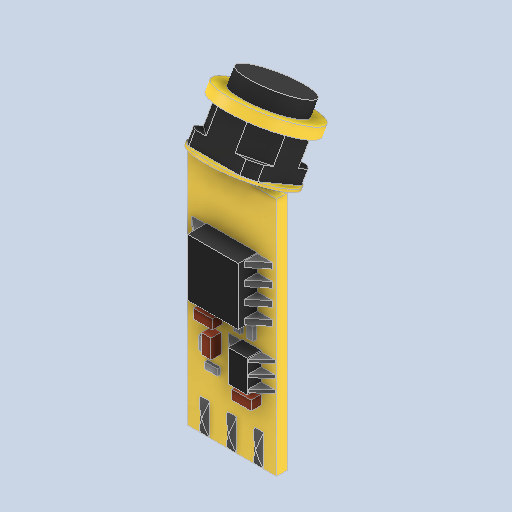
# Autodesk Inventor part: PScaled Modelart2
Saved by Autodesk Inventor 2026.2 (Build 302298010, 298A)
## iProperties
Created: 2026-05-05
Part Number: PScaled Modelart2
Material: Generic
Document SubType Name: Modeling
Designer: piete
Density: 1 g/cm^3
Appearance: Gray
Author: piete
Autodesk Inventor part; units mm, degrees
sketch "Sketch1" plane through (0, 0, 0) normal (1, 0, 0) x (0, 1, 0)
  line L0 (10.261, 0.445) -> (-8.629, 0.445)
  line L1 (-8.629, 0.445) -> (-8.629, -0.445)
  line L2 (-8.629, -0.445) -> (10.261, -0.445)
  line L3 (10.261, -0.445) -> (10.261, 0.445)
  point P0 (0, 0)
  dimension "d0" = 18.89
  dimension "d1" = 0.89
  dimension "d2" = 0.445
  dimension "d3" = 8.629
  constraints: 8 end point, 2 parallel, 1 horizontal, 1 perpendicular
  measures "d0" distance of L2.end L1.end
  measures "d1" distance of L0.end L1.end
  measures "d2" distance from line of point (0, 0) L2
  measures "d3" distance from line of L1 point (0, 0)
extrude "Extrusion1" add sketch "Sketch1" along normal blind 7
sketch "Sketch7" plane through (0, -8.629, 0.445) normal (0, 0, 1) x (1, 0, 0)
  line L0 (1.5, 14.5) -> (5.5, 14.5)
  line L1 (5.5, 14.5) -> (5.5, 10)
  line L2 (5.5, 10) -> (1.5, 10)
  line L3 (1.5, 10) -> (1.5, 14.5)
  line L4 (7, 18.89) -> (7, 0) projected
  line L5 (0, 0) -> (7, 0) projected
  point P0 (0, 8.629)
  dimension "d55" = 4
  dimension "d56" = 1.5
  dimension "d57" = 10
  dimension "d58" = 4.5
  constraints: 8 end point, 2 parallel, 1 horizontal, 1 perpendicular
  measures "d55" distance of L0.start L0.end
  measures "d56" distance between parallel lines of L4 L1
  measures "d57" distance between parallel lines of L5 L2
  measures "d58" distance of L0.end L1.end
extrude "Extrusion7" add sketch "Sketch7" along normal blind 1.5
sketch "Sketch8" plane through (1.5, 5.871, 0.445) normal (0, 1, 0) x (1, 0, 0)
  line L0 (-1.5, 0) -> (5.5, 0) projected
  line L1 (0, 0) -> (-1.2, 0)
  line L2 (0, 0) -> (0, -1)
  line L3 (0, -1) -> (-1.2, 0)
  line L4 (-1.5, 0.89) -> (-1.5, 0) projected
  point P0 (-1.5, 0.445)
  dimension "d61" = 1.2
  dimension "d62" = 1
  dimension "d63" = 0.3
  constraints: 6 end point, 2 point on line, 1 perpendicular
  measures "d61" distance of L1.start L1.end
  measures "d62" distance of L1.start L2.end
  measures "d63" distance from line of L4 L1.end
extrude "Extrusion8" add sketch "Sketch8" against normal up to surface (4.5 mm away)
sketch "Sketch9" plane through (0, -8.629, 1.945) normal (0, 0, 1) x (1, 0, 0)
  line L0 (0.3, 10) -> (0.3, 14.5) projected
  line L1 (1.5, 14.5) -> (1.5, 10) projected
  line L2 (0.3, 14.5) -> (1.5, 14.5)
  line L3 (1.5, 14.5) -> (1.5, 14.425)
  line L4 (1.5, 14.425) -> (0.3, 14.425)
  line L5 (0.3, 14.425) -> (0.3, 14.5)
  line L6 (0.3, 13.975) -> (1.5, 13.975)
  line L7 (1.5, 13.975) -> (1.5, 13.125)
  line L8 (1.5, 13.125) -> (0.3, 13.125)
  line L9 (0.3, 13.125) -> (0.3, 13.975)
  line L10 (0.3, 12.675) -> (1.5, 12.675)
  line L11 (1.5, 12.675) -> (1.5, 11.825)
  line L12 (1.5, 11.825) -> (0.3, 11.825)
  line L13 (0.3, 11.825) -> (0.3, 12.675)
  line L14 (0.3, 11.375) -> (1.5, 11.375)
  line L15 (1.5, 11.375) -> (1.5, 10.525)
  line L16 (1.5, 10.525) -> (0.3, 10.525)
  line L17 (0.3, 10.525) -> (0.3, 11.375)
  line L18 (0.3, 10) -> (1.5, 10) projected
  line L19 (0.3, 10.075) -> (1.5, 10.075)
  line L20 (1.5, 10.075) -> (1.5, 10)
  line L21 (1.5, 10) -> (0.3, 10)
  line L22 (0.3, 10) -> (0.3, 10.075)
  point P0 (0, 8.629)
  point P1 (0.3, 11.825)
  dimension "d66" = 1.2
  dimension "d67" = 1.2
  dimension "d68" = 1.2
  dimension "d69" = 0.075
  dimension "d70" = 0.075
  dimension "d71" = 0.45
  dimension "d72" = 0.45
  dimension "d73" = 0.45
  dimension "d74" = 0.45
  dimension "d75" = 0.85
  dimension "d76" = 0.85
  constraints: 40 end point, 10 parallel, 5 horizontal, 5 perpendicular, 5 point on line
  measures "d66" distance of L7.end L8.end
  measures "d67" distance of L11.end L12.end
  measures "d68" distance of L15.end L16.end
  measures "d69" distance between parallel lines of L18 L19
  measures "d70" distance between parallel lines of L2 L4
  measures "d71" distance between parallel lines of L4 L6
  measures "d72" distance between parallel lines of L10 L8
  measures "d73" distance between parallel lines of L14 L12
  measures "d74" distance between parallel lines of L19 L16
  measures "d75" distance between parallel lines of L8 L6
  measures "d76" distance between parallel lines of L12 L10
extrude "Extrusion9" cut sketch "Sketch9" against normal up to surface (1.5 mm away) contours L0 L19 L1 L18 | L0 L14 L1 L16 | L0 L10 L1 L12 | L0 L6 L1 L8 | L0 L2 L1 L4
ref_plane "Work Plane1" through (3.5, 0, 0) normal (-1, 0, 0) x (0, 0, 1)
mirror "Mirror1" about plane through (3.5, 0, 0) normal (-1, 0, 0) of "Extrusion8", "Extrusion9"
sketch "Sketch10" plane through (0, -8.629, 0.445) normal (0, 0, 1) x (1, 0, 0)
  line L0 (4.3, 5.5) -> (5.8, 5.5)
  line L1 (5.8, 5.5) -> (5.8, 8)
  line L2 (5.8, 8) -> (4.3, 8)
  line L3 (4.3, 8) -> (4.3, 5.5)
  line L4 (7, 18.89) -> (7, 0) projected
  line L5 (1.5, 10) -> (5.5, 10) projected
  point P0 (0, 8.629)
  dimension "d79" = 1.5
  dimension "d80" = 2.5
  dimension "d81" = 1.2
  dimension "d82" = 2
  constraints: 8 end point, 2 parallel, 1 horizontal, 1 perpendicular
  measures "d79" distance of L2.end L1.end
  measures "d80" distance of L1.end L0.end
  measures "d81" distance between parallel lines of L4 L1
  measures "d82" distance between parallel lines of L5 L2
extrude "Extrusion10" add sketch "Sketch10" along normal blind 1.1
sketch "Sketch11" plane through (4.3, -3.129, 0.445) normal (0, -1, 0) x (1, 0, 0)
  line L0 (1.5, 0) -> (1.5, 1.1) projected
  line L1 (1.5, 0) -> (2.6, 0)
  line L2 (1.2, 0) -> (2.4, 0) projected
  line L3 (1.5, 0) -> (2.6, 0) construction
  line L4 (1.5, 0) -> (1.5, 1)
  line L5 (1.5, 1) -> (2.6, 0)
  point P0 (-4.3, -0.445)
  point P1 (2.6, 0)
  dimension "d85" = 1.1
  dimension "d86" = 0
  dimension "d87" = 1
  constraints: 8 end point, 2 collinear, 1 horizontal, 1 point on line
  measures "d85" distance of L0.start L1.end
  measures "d86" distance between parallel lines of L1 L3
  measures "d87" distance of L0.start L4.end
extrude "Extrusion11" add sketch "Sketch11" against normal up to surface (2.5 mm away)
sketch "Sketch12" plane through (0, -8.629, 1.545) normal (0, 0, 1) x (1, 0, 0)
  line L0 (5.8, 5.5) -> (5.8, 8) projected
  line L1 (5.8, 7.9) -> (6.9, 7.9)
  line L2 (6.9, 7.9) -> (6.9, 7.65)
  line L3 (6.9, 7.65) -> (5.8, 7.65)
  line L4 (5.8, 7.65) -> (5.8, 7.9)
  line L5 (5.8, 6.875) -> (6.9, 6.875)
  line L6 (6.9, 6.875) -> (6.9, 6.625)
  line L7 (6.9, 6.625) -> (5.8, 6.625)
  line L8 (5.8, 6.625) -> (5.8, 6.875)
  line L9 (5.8, 5.85) -> (6.9, 5.85)
  line L10 (6.9, 5.85) -> (6.9, 5.6)
  line L11 (6.9, 5.6) -> (5.8, 5.6)
  line L12 (5.8, 5.6) -> (5.8, 5.85)
  line L13 (6.9, 5.5) -> (5.8, 5.5) projected
  line L14 (6.9, 8) -> (5.8, 8) projected
  line L15 (4.3, 5.5) -> (5.8, 5.5) projected
  line L16 (6.9, 8) -> (6.9, 5.5) projected
  line L17 (5.8, 8) -> (6.9, 8)
  line L18 (6.9, 8) -> (6.9, 5.5)
  line L19 (6.9, 5.5) -> (5.8, 5.5)
  line L20 (5.8, 5.5) -> (5.8, 8)
  point P0 (0, 8.629)
  point P1 (6.9, 6.75)
  dimension "d90" = 1.1
  dimension "d91" = 0.25
  dimension "d92" = 1.1
  dimension "d93" = 0.25
  dimension "d94" = 1.1
  dimension "d95" = 0.25
  dimension "d96" = 0.1
  dimension "d97" = 0.1
  dimension "d98" = 1.25
  constraints: 32 end point, 8 parallel, 4 horizontal, 4 perpendicular, 3 point on line, 1 midpoint, 1 other
  measures "d90" distance of L2.end L3.end
  measures "d91" distance of L1.end L2.end
  measures "d92" distance of L6.end L7.end
  measures "d93" distance of L5.end L6.end
  measures "d94" distance of L10.end L11.end
  measures "d95" distance of L9.end L10.end
  measures "d96" distance between parallel lines of L13 L11
  measures "d97" distance between parallel lines of L14 L1
  measures "d98" distance from line of L15 point (6.9, 6.75)
extrude "Extrusion12" cut sketch "Sketch12" against normal up to surface (1.1 mm away) contours L0 L11 L16 L13 | L0 L7 L16 L9 | L0 L3 L16 L5 | L0 L14 L16 L1
ref_plane "Work Plane2" through (5.05, -3.129, 1.545) normal (1, 0, 0) x (0, 0, -1)
mirror "Mirror2" about plane through (5.05, -3.129, 1.545) normal (1, 0, 0) of "Extrusion11", "Extrusion12"
sketch "Sketch13" plane through (0, -8.629, 0.445) normal (0, 0, 1) x (1, 0, 0)
  line L0 (4.9, 9.5) -> (5.4, 9.5)
  line L1 (5.4, 9.5) -> (5.4, 8.5)
  line L2 (5.4, 8.5) -> (4.9, 8.5)
  line L3 (4.9, 8.5) -> (4.9, 9.5)
  line L4 (3.9, 9.5) -> (4.4, 9.5)
  line L5 (4.4, 9.5) -> (4.4, 8.5)
  line L6 (4.4, 8.5) -> (3.9, 8.5)
  line L7 (3.9, 8.5) -> (3.9, 9.5)
  line L8 (1.1, 6.8) -> (1.6, 6.8)
  line L9 (1.6, 6.8) -> (1.6, 5.8)
  line L10 (1.6, 5.8) -> (1.1, 5.8)
  line L11 (1.1, 5.8) -> (1.1, 6.8)
  line L12 (1.6, 5.25) -> (2.6, 5.25)
  line L13 (2.6, 5.25) -> (2.6, 4.75)
  line L14 (2.6, 4.75) -> (1.6, 4.75)
  line L15 (1.6, 4.75) -> (1.6, 5.25)
  line L16 (5.5, 10) -> (5.5, 14.5) projected
  line L17 (5.8, 8) -> (4.3, 8) projected
  line L18 (1.5, 14.5) -> (1.5, 10) projected
  line L19 (1.5, 10) -> (5.5, 10) projected
  line L20 (4.3, 5.5) -> (5.8, 5.5) projected
  point P0 (0, 8.629)
  point P1 (5.4, 9)
  point P2 (1.35, 6.8)
  dimension "d101" = 0.5
  dimension "d102" = 1
  dimension "d103" = 0.5
  dimension "d104" = 1
  dimension "d105" = 0.5
  dimension "d106" = 1
  dimension "d107" = 1
  dimension "d108" = 0.5
  dimension "d109" = 0.1
  dimension "d110" = 0.5
  dimension "d111" = 0.5
  dimension "d112" = 0.1
  dimension "d113" = 3.2
  dimension "d114" = 0.1
  dimension "d115" = 0.25
  constraints: 32 end point, 8 parallel, 4 horizontal, 4 perpendicular, 2 midpoint, 1 point on line
  measures "d101" distance of L1.end L2.end
  measures "d102" distance of L0.end L1.end
  measures "d103" distance of L5.end L6.end
  measures "d104" distance of L4.end L5.end
  measures "d105" distance of L9.end L10.end
  measures "d106" distance of L8.end L9.end
  measures "d107" distance of L13.end L14.end
  measures "d108" distance of L12.end L13.end
  measures "d109" distance from line of L16 point (5.4, 9)
  measures "d110" distance between parallel lines of L5 L3
  measures "d111" distance between parallel lines of L17 L2
  measures "d112" distance between parallel lines of L9 L18
  measures "d113" distance from line of point (1.35, 6.8) L19
  measures "d114" distance between parallel lines of L18 L15
  measures "d115" distance between parallel lines of L12 L20
extrude "Extrusion13" add sketch "Sketch13" along normal blind 0.25
sketch "Sketch14" plane through (0, -8.629, 0.445) normal (0, 0, 1) x (1, 0, 0)
  line L0 (4.3, 5) -> (5.8, 5)
  line L1 (5.8, 5) -> (5.8, 4.25)
  line L2 (5.8, 4.25) -> (4.3, 4.25)
  line L3 (4.3, 4.25) -> (4.3, 5)
  line L4 (1.25, 9) -> (2.75, 9)
  line L5 (2.75, 9) -> (2.75, 8.25)
  line L6 (2.75, 8.25) -> (1.25, 8.25)
  line L7 (1.25, 8.25) -> (1.25, 9)
  line L8 (1.9, 7.65) -> (2.65, 7.65)
  line L9 (2.65, 7.65) -> (2.65, 6.15)
  line L10 (2.65, 6.15) -> (1.9, 6.15)
  line L11 (1.9, 6.15) -> (1.9, 7.65)
  line L12 (4.3, 5.5) -> (5.8, 5.5) projected
  line L13 (4.3, 8) -> (4.3, 5.5) projected
  line L14 (3.2, 7.65) -> (4.3, 7.65) projected
  line L15 (1.6, 5.8) -> (1.6, 6.8) projected
  line L16 (1.5, 14.5) -> (1.5, 10) projected
  line L17 (1.1, 6.8) -> (1.1, 5.8) projected
  line L18 (1.5, 10) -> (5.5, 10) projected
  point P0 (0, 8.629)
  dimension "d118" = 1.5
  dimension "d119" = 0.75
  dimension "d120" = 1.5
  dimension "d121" = 0.75
  dimension "d122" = 0.75
  dimension "d123" = 1.5
  dimension "d124" = 0.5
  dimension "d125" = 0
  dimension "d126" = 0
  dimension "d127" = 0.3
  dimension "d129" = 0.15
  dimension "d130" = 1
  constraints: 24 end point, 6 parallel, 3 horizontal, 3 perpendicular
  measures "d118" distance of L1.end L2.end
  measures "d119" distance of L0.end L1.end
  measures "d120" distance of L5.end L6.end
  measures "d121" distance of L4.end L5.end
  measures "d122" distance of L9.end L10.end
  measures "d123" distance of L8.end L9.end
  measures "d124" distance between parallel lines of L12 L0
  measures "d125" distance between parallel lines of L13 L3
  measures "d126" distance between parallel lines of L14 L8
  measures "d127" distance between parallel lines of L11 L15
  measures "d129" distance between parallel lines of L7 L17
  measures "d130" distance between parallel lines of L18 L4
extrude "Extrusion14" add sketch "Sketch14" along normal blind 0.8
sketch "Sketch15" plane through (0, -8.629, -0.445) normal (0, -1, 0) x (1, 0, 0)
  line L0 (0, 0.89) -> (7, 0.89) projected
  arc A0 (1.75, 0.89) -> (1, 0.89) centre (1.375, 0.7508) ccw
  line L1 (1, 0.89) -> (1.75, 0.89)
  line L2 (5.5, 0.89) -> (6.7, 0.89) projected
  arc A1 (6, 0.89) -> (5.25, 0.89) centre (5.625, 0.7508) ccw
  arc A2 (3.875, 0.89) -> (3.125, 0.89) centre (3.5, 0.7508) ccw
  point P0 (0, 0.445)
  point P1 (3.5, 0.89)
  point P2 (5.25, 0.89)
  dimension "d133" = 0.75
  dimension "d134" = 0.4
  dimension "d135" = 1
  dimension "d136" = 0.75
  dimension "d137" = 0.4
  dimension "d138" = 1
  dimension "d139" = 0.75
  dimension "d140" = 0.4
  dimension "d141" = 0.375
  constraints: 6 point on circle, 3 centre point, 2 end point, 1 horizontal, 1 point on line, 7 other
  measures "d133" distance of L1.start L1.end
  measures "d134" radius of A0
  measures "d135" distance of point (0, 0.89) L1.start
  measures "d136" distance of A1.start A1.end
  measures "d137" radius of A1
  measures "d138" distance of point (7, 0.89) A1.start
  measures "d139" distance of A2.start A2.end
  measures "d140" radius of A2
  measures "d141" distance of A2.start point (3.5, 0.89)
extrude "Extrusion15" add sketch "Sketch15" against normal blind 2.5
sketch "Sketch16" plane through (7, 0, 0) normal (1, 0, 0) x (0, 0, -1)
  line L0 (-0.445, -6.129) -> (-0.445, -8.629) projected
  line L1 (-0.445, -8.629) -> (0.445, -8.629) projected
  arc A0 (-0.445, -6.129) -> (-0.445, -8.629) centre (2.4201, -7.379) ccw
  line L2 (-0.7058, -8.629) -> (-0.445, -8.629) projected
  line L3 (-0.445, -8.629) -> (-0.7058, -8.629)
  line L4 (-0.7058, -8.629) -> (-0.7058, -6.129)
  line L5 (-0.7058, -8.629) -> (-0.7058, -6.129) projected
  line L6 (-0.445, -6.129) -> (-0.7058, -6.129) projected
  line L7 (-0.7058, -6.129) -> (-0.445, -6.129)
  point P0 (0, 0)
  point P1 (-0.7058, -7.379)
  dimension "d144" = 0
  constraints: 6 end point, 2 collinear, 2 point on circle, 1 centre point, 1 point on line
  measures "d144" distance edge to line of A0 L4
extrude "Extrusion16" cut sketch "Sketch16" against normal through all contours A0 L4 L6 | L2 L4 A0
sketch "Sketch17" plane through (0, -8.629, -0.445) normal (0, 0, -1) x (-1, 0, 0)
  line L0 (-4.6, 10) -> (-2.4, 10)
  line L1 (-2.4, 10) -> (-2.4, 5)
  line L2 (-2.4, 5) -> (-4.6, 5)
  line L3 (-4.6, 5) -> (-4.6, 10)
  line L4 (-7, 0) -> (-7, 18.89) projected
  line L5 (0, 0) -> (-7, 0) projected
  point P0 (0, 8.629)
  dimension "d147" = 2.2
  dimension "d148" = 5
  dimension "d149" = 2.4
  dimension "d150" = 5
  constraints: 8 end point, 2 parallel, 1 horizontal, 1 perpendicular
  measures "d147" distance of L1.end L2.end
  measures "d148" distance of L0.end L1.end
  measures "d149" distance between parallel lines of L4 L3
  measures "d150" distance between parallel lines of L5 L2
extrude "Extrusion17" add sketch "Sketch17" along normal blind 0.6
sketch "Sketch18" plane through (0, -8.629, -0.445) normal (0, 0, -1) x (-1, 0, 0)
  line L0 (-6, 14) -> (-5.6, 14)
  line L1 (-5.6, 14) -> (-5.6, 13)
  line L2 (-5.6, 13) -> (-6, 13)
  line L3 (-6, 13) -> (-6, 14)
  line L4 (-6, 12) -> (-5.6, 12)
  line L5 (-5.6, 12) -> (-5.6, 11)
  line L6 (-5.6, 11) -> (-6, 11)
  line L7 (-6, 11) -> (-6, 12)
  line L8 (-2, 4.5) -> (-1, 4.5)
  line L9 (-1, 4.5) -> (-1, 4.1)
  line L10 (-1, 4.1) -> (-2, 4.1)
  line L11 (-2, 4.1) -> (-2, 4.5)
  line L12 (0, 0) -> (0, 18.89) projected
  line L13 (-4.6, 5) -> (-2.4, 5) projected
  line L14 (-7, 0) -> (-7, 18.89) projected
  line L15 (-2.4, 10) -> (-4.6, 10) projected
  point P0 (0, 8.629)
  dimension "d153" = 0.4
  dimension "d154" = 1
  dimension "d155" = 0.4
  dimension "d156" = 1
  dimension "d157" = 1
  dimension "d158" = 0.4
  dimension "d159" = 1
  dimension "d160" = 0.5
  dimension "d161" = 1
  dimension "d162" = 1
  dimension "d163" = 1
  dimension "d164" = 1
  constraints: 24 end point, 6 parallel, 3 horizontal, 3 perpendicular
  measures "d153" distance of L1.end L2.end
  measures "d154" distance of L0.end L1.end
  measures "d155" distance of L5.end L6.end
  measures "d156" distance of L4.end L5.end
  measures "d157" distance of L9.end L10.end
  measures "d158" distance of L8.end L9.end
  measures "d159" distance between parallel lines of L12 L9
  measures "d160" distance between parallel lines of L8 L13
  measures "d161" distance between parallel lines of L14 L7
  measures "d162" distance between parallel lines of L14 L3
  measures "d163" distance between parallel lines of L4 L2
  measures "d164" distance between parallel lines of L15 L6
extrude "Extrusion18" add sketch "Sketch18" along normal blind 0.3
sketch "Sketch19" plane through (0, -8.629, -0.445) normal (0, 0, -1) x (-1, 0, 0)
  line L0 (-1.25, 6.5) -> (-0.75, 6.5)
  line L1 (-0.75, 6.5) -> (-0.75, 5.2)
  line L2 (-0.75, 5.2) -> (-1.25, 5.2)
  line L3 (-1.25, 5.2) -> (-1.25, 6.5)
  line L4 (-1.25, 8.8) -> (-0.75, 8.8)
  line L5 (-0.75, 8.8) -> (-0.75, 7.5)
  line L6 (-0.75, 7.5) -> (-1.25, 7.5)
  line L7 (-1.25, 7.5) -> (-1.25, 8.8)
  line L8 (-5.8, 5.6) -> (-6.9, 5.6) projected
  line L9 (-6.25, 5.6) -> (-5.75, 5.6)
  line L10 (-5.75, 5.6) -> (-5.75, 6.9)
  line L11 (-5.75, 6.9) -> (-6.25, 6.9)
  line L12 (-6.25, 6.9) -> (-6.25, 5.6)
  line L13 (-2.4, 11.5) -> (-1.1, 11.5)
  line L14 (-1.1, 11.5) -> (-1.1, 11)
  line L15 (-1.1, 11) -> (-2.4, 11)
  line L16 (-2.4, 11) -> (-2.4, 11.5)
  line L17 (0, 0) -> (0, 18.89) projected
  line L18 (-4.6, 5) -> (-2.4, 5) projected
  line L19 (-6.25, 10.3) -> (-5.75, 10.3)
  line L20 (-5.75, 10.3) -> (-5.75, 9)
  line L21 (-5.75, 9) -> (-6.25, 9)
  line L22 (-6.25, 9) -> (-6.25, 10.3)
  line L23 (-2.4, 10) -> (-4.6, 10) projected
  line L24 (-7, 0) -> (-7, 18.89) projected
  line L25 (-2.4, 5) -> (-2.4, 10) projected
  point P0 (0, 8.629)
  dimension "d167" = 0.5
  dimension "d168" = 1.3
  dimension "d169" = 0.5
  dimension "d170" = 1.3
  dimension "d171" = 0.5
  dimension "d172" = 1.3
  dimension "d175" = 1.3
  dimension "d176" = 0.5
  dimension "d177" = 0.75
  dimension "d178" = 0.2
  dimension "d179" = 1
  dimension "d180" = 0.5
  dimension "d181" = 1.3
  dimension "d182" = 0.3
  dimension "d183" = 0.75
  dimension "d184" = 0.75
  dimension "d185" = 0
  dimension "d186" = 1
  constraints: 40 end point, 10 parallel, 5 horizontal, 5 perpendicular, 2 point on line
  measures "d167" distance of L1.end L2.end
  measures "d168" distance of L0.end L1.end
  measures "d169" distance of L5.end L6.end
  measures "d170" distance of L4.end L5.end
  measures "d171" distance of L11.end L10.end
  measures "d172" distance of L10.end L9.end
  measures "d175" distance of L14.end L15.end
  measures "d176" distance of L13.end L14.end
  measures "d177" distance between parallel lines of L17 L1
  measures "d178" distance between parallel lines of L18 L2
  measures "d179" distance between parallel lines of L6 L0
  measures "d180" distance of L20.end L21.end
  measures "d181" distance of L19.end L20.end
  measures "d182" distance from line of L19.end L23
  measures "d183" distance between parallel lines of L24 L22
  measures "d184" distance between parallel lines of L12 L24
  measures "d185" distance between parallel lines of L25 L16
  measures "d186" distance between parallel lines of L23 L15
extrude "Extrusion19" add sketch "Sketch19" along normal blind 0.6
mirror "Mirror3" about plane through (0, 0, 0) normal (0, 0, 1) of "Extrusion15", "Extrusion16"
ref_plane "Work Plane4" through (0, 10.261, -0.445) normal (0, 0.8660254, -0.5) x (1, 0, 0)
sketch "Sketch20" plane through (0, 10.261, -0.445) normal (0, 0.8660254, -0.5) x (1, 0, 0)
  line L0 (0, 0) -> (7, 0) projected
  circle A0 centre (3.5, 0) radius 3.5
  line L1 (0, 9.445) -> (0, 0) projected
  point P0 (0, 4.7451)
  constraints: 1 centre point, 1 midpoint, 1 tangent
extrude "Extrusion20" add sketch "Sketch20" along normal blind 0.2
sketch "Sketch21" plane through (3.5, 10.4342, -0.545) normal (0, 0.8660254, -0.5) x (1, 0, 0)
  circle A0 centre (0, 0) radius 2.5
  line L0 (-3.5, 9.445) -> (-3.5, 0) projected
  circle A1 centre (0, 0) radius 3.5 projected
  point P0 (-3.5, 4.7451)
  dimension "d192" = 5
  dimension "d193" = 3.5
  dimension "d194" = 1
  constraints: 1 centre point, 1 horizontal alignment
  measures "d192" diameter of A0
  measures "d193" distance from line of L0 A0.centre
extrude "Extrusion21" add sketch "Sketch21" along normal blind 5 contours A0
sketch "Sketch22" plane through (3.5, 10.4342, -0.545) normal (0, 0.8660254, -0.5) x (1, 0, 0)
  line L0 (2.75, -2.75) -> (-2.75, -2.75)
  line L1 (-2.75, -2.75) -> (-2.75, 2.75)
  line L2 (-2.75, 2.75) -> (2.75, 2.75)
  line L3 (2.75, 2.75) -> (2.75, -2.75)
  circle A0 centre (0, 0) radius 3.5 projected
  circle A1 centre (0, 0) radius 2.5 projected
  circle A2 centre (0, 0) radius 3.4
  point P0 (-3.5, 4.7451)
  point P1 (-1.9994, 2.75)
  point P2 (-2.75, 1.9994)
  point P3 (-2.75, -1.9994)
  point P4 (-1.9994, -2.75)
  point P5 (1.9994, -2.75)
  point P6 (2.75, -1.9994)
  point P7 (2.75, 1.9994)
  point P8 (1.9994, 2.75)
  dimension "d197" = 0.75
  dimension "d198" = 0.75
  dimension "d199" = 0.75
  dimension "d200" = 0.75
  dimension "d201" = 6.8
  constraints: 8 end point, 2 parallel, 1 centre point, 1 coincident, 1 horizontal, 1 perpendicular
  measures "d197" distance edge to line of A0 L2
  measures "d198" distance edge to line of A0 L0
  measures "d199" distance edge to line of A0 L1
  measures "d200" distance edge to line of A0 L3
  measures "d201" diameter of A2
extrude "Extrusion22" add sketch "Sketch22" along normal blind 1 contours L0 A2 L1 L2 L3
sketch "Sketch23" plane through (3.5, 11.3002, -1.045) normal (0, 0.8660254, -0.5) x (1, 0, 0)
  line L0 (-2.75, 1.1391) -> (-1.1391, 2.75)
  line L1 (-1.1391, 2.75) -> (1.1391, 2.75)
  line L2 (1.1391, 2.75) -> (2.75, 1.1391)
  line L3 (2.75, 1.1391) -> (2.75, -1.1391)
  line L4 (2.75, -1.1391) -> (1.1391, -2.75)
  line L5 (1.1391, -2.75) -> (-1.1391, -2.75)
  line L6 (-1.1391, -2.75) -> (-2.75, -1.1391)
  line L7 (-2.75, -1.1391) -> (-2.75, 1.1391)
  line L8 (-1.9994, -2.75) -> (1.9994, -2.75) projected
  line L9 (1.9994, 2.75) -> (-1.9994, 2.75) projected
  line L10 (2.75, -1.9994) -> (2.75, 1.9994) projected
  point P0 (-3.5, 4.7451)
  point P1 (0, 0)
  constraints: 16 end point, 3 collinear, 17 other
extrude "Extrusion23" add sketch "Sketch23" along normal blind 2
sketch "Sketch24" plane through (3.5, 13.0323, -2.045) normal (0, 0.8660254, -0.5) x (1, 0, 0)
  line L0 (-3.5, 0) -> (3.5, 0) projected
  circle A0 centre (0, 0) radius 3.5
  circle A1 centre (0, 0) radius 2.5
  point P0 (-3.5, 4.7451)
  dimension "d206" = 7
  constraints: 2 centre point, 1 coincident, 1 midpoint
  measures "d206" diameter of A0
extrude "Extrusion24" add sketch "Sketch24" along normal blind 0.8 contours A1 L0 A0 | L0 A0 A1
ref_plane "Work Plane3" through (0, 0, 0) normal (0, 0, 1) x (1, 0, 0)
equation "\"d2\" = 0.5 * d1"
equation "\"d141\" = 0.5 * d139"
body "Solid1"
